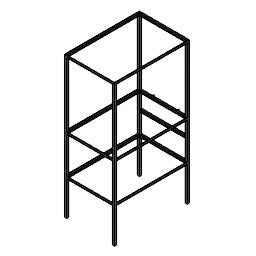
Shelf (Autodesk Fusion 360 design; units mm, degrees)
part number: 2026-04-06-11-05-22-713
Autodesk Fusion 360 part; units mm, degrees
note: some values were not read from the file. Set by a fixed rule: which sketch regions a step uses.
sketch "Sketch1" plane through (0, 0, 0) normal (0, 0, 1) x (1, 0, 0)
  line L0 (0, 0) -> (25.4, 0)
  line L1 (25.4, 0) -> (25.4, 25.4)
  line L2 (25.4, 25.4) -> (0, 25.4)
  line L3 (0, 25.4) -> (0, 0)
  dimension "d1" = 25.4
  dimension "d2" = 25.4
  constraint horizontal L0
  constraint vertical L1
  constraint horizontal L2
  constraint vertical L3
  constraint coincident L0.start L3.end
  measures "d1" distance of L0.start L0.end
  measures "d2" distance of L0.start L2.end
extrude "Extrude1" add sketch "Sketch1" along normal blind 914.4 makes body 1
sketch "Sketch2" plane through (0, 0, 914.4) normal (0, 0, 1) x (1, 0, 0)
  line L0 (0, 25.4) -> (0, 0)
  line L1 (0, 0) -> (25.4, 0)
  line L2 (25.4, 0) -> (25.4, 25.4)
  line L3 (25.4, 25.4) -> (0, 25.4)
  line L4 (0, 0) -> (609.6, 0)
  line L5 (609.6, 0) -> (609.6, 914.4)
  line L6 (609.6, 914.4) -> (0, 914.4)
  line L7 (0, 914.4) -> (0, 0)
  dimension "d5" = 609.6
  dimension "d6" = 914.4
  constraint horizontal L4
  constraint vertical L5
  constraint horizontal L6
  constraint vertical L7
  constraint coincident L0.end L1.start
  measures "d5" distance of L0.end L4.end
  measures "d6" distance of L0.end L6.end
sketch "Sketch3" plane through (0, 0, 914.4) normal (0, 0, 1) x (1, 0, 0)
  line L0 (0, 914.4) -> (25.4, 914.4)
  line L1 (25.4, 914.4) -> (25.4, 889)
  line L2 (25.4, 889) -> (0, 889)
  line L3 (0, 889) -> (0, 914.4)
  line L4 (609.6, 914.4) -> (0, 914.4)
  line L5 (0, 914.4) -> (0, 0)
  line L6 (609.6, 914.4) -> (584.2, 914.4)
  line L7 (584.2, 914.4) -> (584.2, 889)
  line L8 (584.2, 889) -> (609.6, 889)
  line L9 (609.6, 889) -> (609.6, 914.4)
  line L10 (609.6, 0) -> (609.6, 914.4)
  line L11 (609.6, 0) -> (584.2, 0)
  line L12 (584.2, 0) -> (584.2, 25.4)
  line L13 (584.2, 25.4) -> (609.6, 25.4)
  line L14 (609.6, 25.4) -> (609.6, 0)
  line L15 (0, 0) -> (609.6, 0)
  dimension "d7" = 25.4
  dimension "d8" = 25.4
  dimension "d9" = 25.4
  dimension "d10" = 25.4
  dimension "d11" = 25.4
  dimension "d12" = 25.4
  constraint horizontal L0
  constraint vertical L1
  constraint horizontal L2
  constraint vertical L3
  constraint collinear L0 L4
  constraint collinear L3 L5
  constraint horizontal L6
  constraint vertical L7
  constraint horizontal L8
  constraint vertical L9
  constraint collinear L4 L6
  constraint collinear L9 L10
  constraint horizontal L11
  constraint vertical L12
  constraint horizontal L13
  constraint vertical L14
  constraint collinear L11 L15
  constraint collinear L10 L14
  measures "d7" distance of L0.start L0.end
  measures "d8" distance of L0.start L2.end
  measures "d9" distance of L4.start L6.end
  measures "d10" distance of L4.start L8.end
  measures "d11" distance of L10.start L11.end
  measures "d12" distance of L10.start L13.end
extrude "Extrude2" add sketch "Sketch3" against normal blind 914.4 separate body contours L0 L1 L2 L3 L4 L5 | L4 L6 L7 L8 L9 L10 | L10 L11 L12 L13 L14 L15 makes body 2 at (25.4, 905.9333, 304.8) makes body 3 at (609.6, 897.4667, 304.8) makes body 4 at (584.2, 8.4667, 304.8)
sketch "Sketch4" plane through (0, 0, 914.4) normal (0, 0, 1) x (1, 0, 0)
  line L0 (584.2, 889) -> (609.6, 889)
  line L1 (609.6, 889) -> (609.6, 25.4)
  line L2 (609.6, 25.4) -> (584.2, 25.4)
  line L3 (584.2, 25.4) -> (584.2, 889)
  line L4 (0, 914.4) -> (584.2, 914.4)
  line L5 (584.2, 914.4) -> (584.2, 889)
  line L6 (584.2, 889) -> (0, 889)
  line L7 (0, 889) -> (0, 914.4)
  line L8 (0, 914.4) -> (25.4, 914.4)
  line L9 (25.4, 914.4) -> (25.4, 0)
  line L10 (25.4, 0) -> (0, 0)
  line L11 (0, 0) -> (0, 914.4)
  line L12 (0, 0) -> (584.2, 0)
  line L13 (584.2, 0) -> (584.2, 25.4)
  line L14 (584.2, 25.4) -> (0, 25.4)
  line L15 (0, 25.4) -> (0, 0)
  line L16 (0, 0) -> (609.6, 0)
  line L17 (0, 914.4) -> (0, 0)
  line L18 (609.6, 914.4) -> (0, 914.4)
  line L19 (609.6, 0) -> (609.6, 914.4)
  line L20 (609.6, 889) -> (609.6, 914.4)
  line L21 (609.6, 914.4) -> (584.2, 914.4)
  dimension "d15" = 25.4
  dimension "d16" = 25.4
  dimension "d17" = 25.4
  dimension "d18" = 25.4
  constraint horizontal L0
  constraint vertical L1
  constraint horizontal L2
  constraint vertical L3
  constraint horizontal L4
  constraint vertical L5
  constraint horizontal L6
  constraint vertical L7
  constraint horizontal L8
  constraint vertical L9
  constraint horizontal L10
  constraint vertical L11
  constraint horizontal L12
  constraint vertical L13
  constraint horizontal L14
  constraint vertical L15
  constraint collinear L8 L18
  constraint collinear L7 L17
  constraint collinear L15 L17
  constraint collinear L10 L16
  constraint collinear L12 L16
  constraint collinear L1 L20
  constraint collinear L4 L21
  constraint collinear L11 L17
  measures "d15" distance of L14 L16
  measures "d16" distance of L9 L17
  measures "d17" distance of L6 L18
  measures "d18" distance of L3 L19
extrude "Extrude3" add sketch "Sketch4" against normal blind 25.4 separate body contours L0 L1 L2 L3 L19 | L4 L5 L6 L9 L18 | L9 L12 L13 L14 L16 | L6 L9 L11 L14 L17 makes body 5 at (397.9333, 897.4667, 914.4)
ref_plane "WorkPlane1" through (596.9, 901.7, 444.5) normal (0, 0, -1) x (-1, 0, 0)
sketch "Sketch5" plane through (0, 0, 444.5) normal (0, 0, -1) x (-1, 0, 0)
  line L0 (-609.6, 1066.8) -> (0, 1066.8)
  line L1 (0, 1066.8) -> (0, 0)
  line L2 (0, 0) -> (-609.6, 0)
  line L3 (-609.6, 0) -> (-609.6, 1066.8)
  line L4 (-584.2, 889) -> (-25.4, 889)
  line L5 (-584.2, 914.4) -> (-584.2, 889)
  line L6 (-584.2, 914.4) -> (-25.4, 914.4)
  line L7 (-25.4, 914.4) -> (-25.4, 889)
  line L8 (-25.4, 889) -> (0, 889)
  line L9 (0, 889) -> (0, 25.4)
  line L10 (-25.4, 25.4) -> (0, 25.4)
  line L11 (-25.4, 889) -> (-25.4, 25.4)
  line L12 (-584.2, 889) -> (-609.6, 889)
  line L13 (-584.2, 25.4) -> (-584.2, 889)
  line L14 (-609.6, 25.4) -> (-584.2, 25.4)
  line L15 (-609.6, 25.4) -> (-609.6, 889)
  line L16 (-25.4, 0) -> (-584.2, 0)
  line L17 (-584.2, 0) -> (-584.2, 25.4)
  line L18 (-584.2, 25.4) -> (-25.4, 25.4)
  line L19 (-25.4, 25.4) -> (-25.4, 0)
  dimension "d22" = 609.6
  dimension "d23" = 1066.8
  constraint horizontal L0
  constraint vertical L1
  constraint horizontal L2
  constraint vertical L3
  constraint coincident L1.end L2.start
  measures "d22" distance of L1 L3
  measures "d23" distance of L0 L2
extrude "Extrude4" add sketch "Sketch5" along normal blind 25.4 separate body contours L3 L12 L13 L14 L15 | L1 L8 L9 L10 L11 | L4 L5 L6 L7 | L2 L16 L17 L18 L19 makes body 6 at (397.9333, 25.4, 436.0333)
ref_plane "WorkPlane2" through (304.8, 901.7, 1727.2) normal (0, 0, 1) x (1, 0, 0)
sketch "Sketch6" plane through (0, 0, 1727.2) normal (0, 0, 1) x (1, 0, 0)
  line L0 (584.2, 889) -> (25.4, 889)
  line L1 (584.2, 914.4) -> (584.2, 889)
  line L2 (25.4, 914.4) -> (584.2, 914.4)
  line L3 (25.4, 889) -> (25.4, 914.4)
  line L4 (0, 889) -> (25.4, 889)
  line L5 (0, 25.4) -> (0, 889)
  line L6 (25.4, 25.4) -> (0, 25.4)
  line L7 (25.4, 889) -> (25.4, 25.4)
  line L8 (584.2, 889) -> (609.6, 889)
  line L9 (584.2, 25.4) -> (584.2, 889)
  line L10 (609.6, 25.4) -> (584.2, 25.4)
  line L11 (609.6, 889) -> (609.6, 25.4)
  line L12 (584.2, 0) -> (25.4, 0)
  line L13 (584.2, 25.4) -> (584.2, 0)
  line L14 (25.4, 25.4) -> (584.2, 25.4)
  line L15 (25.4, 0) -> (25.4, 25.4)
  line L16 (25.4, 25.4) -> (0, 25.4)
  line L17 (25.4, 0) -> (25.4, 25.4)
  line L18 (0, 0) -> (25.4, 0)
  line L19 (0, 25.4) -> (0, 0)
  line L20 (609.6, 25.4) -> (609.6, 0)
  line L21 (584.2, 25.4) -> (609.6, 25.4)
  line L22 (584.2, 0) -> (584.2, 25.4)
  line L23 (609.6, 0) -> (584.2, 0)
  line L24 (609.6, 914.4) -> (609.6, 889)
  line L25 (584.2, 914.4) -> (609.6, 914.4)
  line L26 (584.2, 889) -> (584.2, 914.4)
  line L27 (609.6, 889) -> (584.2, 889)
  line L28 (0, 889) -> (0, 914.4)
  line L29 (25.4, 889) -> (0, 889)
  line L30 (25.4, 914.4) -> (25.4, 889)
  line L31 (0, 914.4) -> (25.4, 914.4)
extrude "Extrude5" add sketch "Sketch6" against normal blind 812.8 contours L1 L8 L24 L25 L26 L27 | L3 L4 L28 L29 L30 L31 | L10 L13 L20 L21 L22 L23 | L6 L15 L16 L17 L18 L19 bodies 1 6 2 3 4 5
extrude "Extrude6" add sketch "Sketch6" against normal blind 25.4 contours L0 L1 L2 L3 L26 L30 | L8 L9 L10 L11 L21 L27 | L4 L5 L6 L7 L16 L29 | L12 L13 L14 L15 L17 L22 bodies 1
combine "Combine1" operation add target body 1 tool bodies 6
sketch "Sketch7" plane through (0, 0, 0) normal (0, -1, 0) x (1, 0, 0)
  line L0 (25.4, 444.5) -> (25.4, 889)
  line L1 (25.4, 889) -> (584.2, 889)
  line L2 (584.2, 889) -> (584.2, 444.5)
  line L3 (584.2, 444.5) -> (25.4, 444.5)
  line L4 (25.4, 419.1) -> (584.2, 419.1)
  line L5 (584.2, 419.1) -> (584.2, 0)
  line L6 (584.2, 0) -> (609.6, 0)
  line L7 (609.6, 0) -> (609.6, 1727.2)
  line L8 (609.6, 1727.2) -> (584.2, 1727.2)
  line L9 (584.2, 1727.2) -> (0, 1727.2)
  line L10 (0, 1727.2) -> (0, 0)
  line L11 (0, 0) -> (25.4, 0)
  line L12 (25.4, 0) -> (25.4, 419.1)
  line L13 (25.4, 1701.8) -> (584.2, 1701.8)
  line L14 (584.2, 1701.8) -> (584.2, 914.4)
  line L15 (584.2, 914.4) -> (25.4, 914.4)
  line L16 (25.4, 914.4) -> (25.4, 1701.8)
  circle A0 centre (457.2, 901.7) radius 6.35
  circle A1 centre (152.4, 901.7) radius 6.35
  line L17 (152.4, 901.7) -> (457.2, 901.7)
  line L18 (152.4, 901.7) -> (152.4, 685.8)
  line L19 (25.4, 711.2) -> (584.2, 711.2)
  line L20 (584.2, 711.2) -> (584.2, 685.8)
  line L21 (584.2, 685.8) -> (25.4, 685.8)
  line L22 (25.4, 685.8) -> (25.4, 711.2)
  dimension "d31" = 12.7
  dimension "d33" = 12.7
  dimension "d34" = 304.8
  dimension "d35" = 152.4
  dimension "d36" = 12.7
  dimension "d37" = 215.9
  dimension "d38" = 25.4
  constraint coincident A1.centre L17.start
  constraint coincident A0.centre L17.end
  constraint horizontal L17
  constraint perpendicular L17 L18
  constraint horizontal L19
  constraint vertical L20
  constraint horizontal L21
  constraint vertical L22
  constraint coincident L2 L20.end
  constraint coincident L0 L19.start
  constraint coincident L18.end L21
  measures "d31" diameter of A0
  measures "d33" diameter of A1
  measures "d34" horizontal distance of A0.centre A1.centre
  measures "d35" distance of L10 A1.centre
  measures "d36" distance of L1 L17
  measures "d37" distance of A1.centre L18.end
  measures "d38" distance of L19 L21
extrude "Extrude7" add sketch "Sketch7" against normal blind 25.4 contours L0 L18 L19 L21 L22 | L2 L18 L19 L20 L21 bodies 1
extrude "Extrude8" add sketch "Sketch7" along normal blind 25.4 contours A0 | A1 L17 L18 | A1 L17 L18 bodies 1
sketch "Sketch8" plane through (0, 0, 1727.2) normal (0, 0, 1) x (1, 0, 0)
  line L0 (0, 914.4) -> (0, 0)
  line L1 (0, 0) -> (584.2, 0)
  line L2 (584.2, 0) -> (609.6, 0)
  line L3 (609.6, 0) -> (609.6, 25.4)
  line L4 (609.6, 25.4) -> (609.6, 889)
  line L5 (609.6, 889) -> (609.6, 914.4)
  line L6 (609.6, 914.4) -> (0, 914.4)
  line L7 (25.4, 25.4) -> (25.4, 889)
  line L8 (25.4, 889) -> (584.2, 889)
  line L9 (584.2, 889) -> (584.2, 25.4)
  line L10 (584.2, 25.4) -> (25.4, 25.4)
  line L11 (6.35, 908.05) -> (603.25, 908.05)
  line L12 (603.25, 908.05) -> (603.25, 6.35)
  line L13 (603.25, 6.35) -> (6.35, 6.35)
  line L14 (6.35, 6.35) -> (6.35, 908.05)
  dimension "d43" = 6.35
  dimension "d44" = 6.35
  dimension "d45" = 6.35
  dimension "d46" = 6.35
  constraint horizontal L11
  constraint vertical L12
  constraint horizontal L13
  constraint vertical L14
  measures "d43" distance of L4 L12
  measures "d44" distance of L1 L13
  measures "d45" distance of L6 L11
  measures "d46" distance of L0 L14
extrude "Extrude9" cut sketch "Sketch8" against normal blind 19.05 contours L11 L12 L13 L14 bodies 1
sketch "Sketch9" plane through (0, 0, 914.4) normal (0, 0, 1) x (1, 0, 0)
  line L0 (25.4, 889) -> (0, 889)
  line L1 (0, 889) -> (0, 25.4)
  line L2 (0, 25.4) -> (25.4, 25.4)
  line L3 (25.4, 25.4) -> (25.4, 889)
  line L4 (6.35, 908.05) -> (603.25, 908.05)
  line L5 (603.25, 908.05) -> (603.25, 6.35)
  line L6 (603.25, 6.35) -> (6.35, 6.35)
  line L7 (6.35, 6.35) -> (6.35, 908.05)
  line L8 (25.4, 914.4) -> (25.4, 889)
  line L9 (25.4, 889) -> (584.2, 889)
  line L10 (584.2, 889) -> (584.2, 914.4)
  line L11 (584.2, 914.4) -> (25.4, 914.4)
  line L12 (584.2, 25.4) -> (609.6, 25.4)
  line L13 (609.6, 25.4) -> (609.6, 889)
  line L14 (609.6, 889) -> (584.2, 889)
  line L15 (584.2, 889) -> (584.2, 25.4)
  line L16 (584.2, 0) -> (584.2, 25.4)
  line L17 (584.2, 25.4) -> (25.4, 25.4)
  line L18 (25.4, 25.4) -> (25.4, 0)
  line L19 (25.4, 0) -> (584.2, 0)
  dimension "d49" = 6.35
  dimension "d50" = 6.35
  dimension "d51" = 6.35
  dimension "d52" = 6.35
  constraint horizontal L4
  constraint vertical L5
  constraint horizontal L6
  constraint vertical L7
  measures "d49" distance of L5 L13
  measures "d50" distance of L6 L19
  measures "d51" distance of L1 L7
  measures "d52" distance of L4 L11
extrude "Extrude10" cut sketch "Sketch9" against normal blind 19.05 contours L0 L2 L3 L7 | L3 L9 L15 L17 | L4 L8 L9 L10 | L6 L16 L17 L18 | L5 L12 L14 L15 bodies 1
sketch "Sketch10" plane through (0, 0, 711.2) normal (0, 0, 1) x (1, 0, 0)
  line L0 (25.4, 0) -> (584.2, 0)
  line L1 (584.2, 0) -> (584.2, 25.4)
  line L2 (584.2, 25.4) -> (25.4, 25.4)
  line L3 (25.4, 25.4) -> (25.4, 0)
  line L4 (15.2621, 59.1079) -> (599.5555, 59.1079)
  line L5 (599.5555, 59.1079) -> (599.5555, 6.35)
  line L6 (599.5555, 6.35) -> (15.2621, 6.35)
  line L7 (15.2621, 6.35) -> (15.2621, 59.1079)
  dimension "d55" = 6.35
  constraint horizontal L4
  constraint vertical L5
  constraint horizontal L6
  constraint vertical L7
  measures "d55" distance of L0 L6
extrude "Extrude11" cut sketch "Sketch10" against normal blind 19.05 contours L1 L2 L3 L6 bodies 1
sketch "Sketch11" plane through (0, 0, 444.5) normal (0, 0, 1) x (1, 0, 0)
  line L0 (584.2, 25.4) -> (25.4, 25.4)
  line L1 (25.4, 25.4) -> (25.4, 0)
  line L2 (25.4, 0) -> (584.2, 0)
  line L3 (584.2, 0) -> (584.2, 25.4)
  line L4 (25.4, 889) -> (0, 889)
  line L5 (0, 889) -> (0, 25.4)
  line L6 (0, 25.4) -> (25.4, 25.4)
  line L7 (25.4, 25.4) -> (25.4, 889)
  line L8 (584.2, 914.4) -> (25.4, 914.4)
  line L9 (584.2, 889) -> (25.4, 889)
  line L10 (609.6, 25.4) -> (609.6, 889)
  line L11 (584.2, 889) -> (584.2, 25.4)
  line L12 (584.2, 25.4) -> (609.6, 25.4)
  line L13 (609.6, 25.4) -> (609.6, 889)
  line L14 (609.6, 889) -> (584.2, 889)
  line L15 (584.2, 889) -> (584.2, 914.4)
  line L16 (584.2, 914.4) -> (25.4, 914.4)
  line L17 (25.4, 914.4) -> (25.4, 889)
  line L18 (25.4, 889) -> (584.2, 889)
  line L19 (6.35, 908.05) -> (603.25, 908.05)
  line L20 (603.25, 908.05) -> (603.25, 6.35)
  line L21 (603.25, 6.35) -> (6.35, 6.35)
  line L22 (6.35, 6.35) -> (6.35, 908.05)
  dimension "d58" = 6.35
  dimension "d59" = 6.35
  dimension "d60" = 6.35
  dimension "d61" = 6.35
  constraint horizontal L19
  constraint vertical L20
  constraint horizontal L21
  constraint vertical L22
  measures "d58" distance of L13 L20
  measures "d59" distance of L2 L21
  measures "d60" distance of L5 L22
  measures "d61" distance of L8 L19
extrude "Extrude12" cut sketch "Sketch11" against normal blind 19.05 contours L0 L1 L3 L21 | L11 L12 L14 L20 | L4 L6 L7 L22 | L9 L15 L17 L18 L19 bodies 1
equation "d21 = ( -35 / 2 ) * 1 in"
equation "d34 = 12.5 in - 0.25 in - 0.25 in"
equation "d43 = ( 1 / 4 ) * 1 in"
equation "d44 = d43"
equation "d45 = d44"
equation "d46 = d44"
equation "d47 = -1 in + d44"
equation "d49 = d44"
equation "d50 = d44"
equation "d51 = d44"
equation "d52 = d44"
equation "d53 = -1 in + d44"
equation "d55 = d44"
equation "d56 = -1 in + d44"
equation "d58 = d44"
equation "d59 = d44"
equation "d60 = d44"
equation "d61 = d44"
equation "d62 = -1 in + d44"
